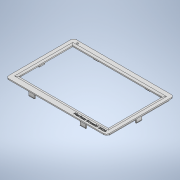
# Autodesk Inventor part: Top
Saved by Autodesk Inventor 2021 (Build 250183000, 183)
## iProperties
Created: 2020-06-15
Part Number: Top
Material: Generic
Document SubType Name: Modeling
Designer: Mariano
Density: 1 g/cm^3
Appearance: Default
Author: Mariano
Autodesk Inventor part; units mm, degrees
ref_plane "YZ Plane" through (0, 0, 0) normal (1, 0, 0) x (0, 1, 0)
ref_plane "XZ Plane" through (0, 0, 0) normal (0, 1, 0) x (-1, 0, 0)
ref_plane "XY Plane" through (0, 0, 0) normal (0, 0, 1) x (1, 0, 0)
sketch "Sketch1" plane through (0, 0, 0) normal (0, 1, 0) x (-1, 0, 0)
  line L0 (-92.2, 62) -> (92.2, 62)
  line L1 (92.2, 62) -> (92.2, -62)
  line L2 (92.2, -62) -> (-92.2, -62)
  line L3 (-92.2, -62) -> (-92.2, 62)
  line L4 (-92.2, 62) -> (92.2, -62) construction
  line L5 (92.2, 62) -> (-92.2, -62) construction
  line L6 (82.2, -50.5) -> (-82.2, -50.5)
  line L7 (-82.2, -50.5) -> (-82.2, 48.5)
  line L8 (-82.2, 48.5) -> (82.2, 48.5)
  line L9 (82.2, 48.5) -> (82.2, -50.5)
  line L10 (82.2, -50.5) -> (-82.2, 48.5) construction
  line L11 (-82.2, -50.5) -> (82.2, 48.5) construction
  line L12 (0, -62) -> (0, 62) construction
  line L13 (129.08, 0) -> (-129.08, 0) projected
  point P0 (0, 0)
  point P1 (0, -50.5)
  dimension "d2" = 184.4
  dimension "d3" = 124
  dimension "d34" = 164.4
  dimension "d35" = 99
  dimension "d50" = 13.5
  constraints: 26 end point, 5 midpoint, 5 perpendicular, 3 parallel, 1 point on line
  measures "d2" distance of L0.start L0.end
  measures "d3" distance of L0.end L1.end
  measures "d34" distance of L7.end L8.end
  measures "d35" distance of L6.end L7.end
  measures "d50" distance between parallel lines of L0 L8
extrude "Extrusion2" add sketch "Sketch1" along normal blind 3 contours L0 L1 L13 L9 L8 L7 L3 | L13 L7 L6 L9 L1 L2 L3
sketch "Sketch2" plane through (0, 0, 0) normal (0, -1, 0) x (1, 0, 0)
  line L0 (92.2, -62) -> (-92.2, -62) projected
  line L1 (-92.2, -62) -> (-92.2, 62) projected
  line L2 (92.2, -62) -> (-92.2, -62)
  line L3 (-92.2, -62) -> (-92.2, 62)
  line L4 (-92.2, 62) -> (92.2, 62)
  line L5 (92.2, 62) -> (92.2, -62)
  line L6 (90.2, -60) -> (-90.2, -60)
  line L7 (-90.2, -60) -> (-90.2, 60)
  line L8 (-90.2, 60) -> (90.2, 60)
  line L9 (90.2, 60) -> (90.2, -60)
  line L10 (0, -60) -> (0, 60)
  line L11 (-90.2, 0) -> (90.2, 0)
  point P0 (0, 0)
  dimension "d23" = 2
  constraints: 20 end point, 4 midpoint, 4 parallel, 2 perpendicular, 1 horizontal, 3 other
  measures "d23" distance between parallel lines of L9 L5
chamfer "Chamfer6" distance 4 distance2 1 1 edges at (-82.2, 3, -1) measured on face at (27.4, 3, 57.5)
chamfer "Chamfer7" distance 4 distance2 1 1 edges at (0, 3, -50.5) measured on face at (27.4, 3, 57.5)
chamfer "Chamfer8" distance 4 distance2 1 1 edges at (0, 3, 48.5) measured on face at (27.4, 3, 57.5)
chamfer "Chamfer9" distance 4 distance2 1 1 edges at (82.2, 3, -1) measured on face at (27.4, 3, 58.8333)
extrude "Extrusion5" cut sketch "Sketch2" against normal blind 1
fillet "Fillet1" radius 5 8 edges at (-92.2, 2, 62) (92.2, 2, 62) (-92.2, 2, -62) (92.2, 2, -62) (-90.2, 0.5, 60) (90.2, 0.5, 60) (90.2, 0.5, -60) (-90.2, 0.5, -60)
sketch "Sketch4" plane through (0, 0, 0) normal (0, -1, 0) x (1, 0, 0)
  line L0 (-85.2, -60) -> (85.2, -60) projected
  line L1 (52.2, -60) -> (42.2, -60)
  line L2 (42.2, -60) -> (42.2, -58)
  line L3 (42.2, -58) -> (52.2, -58)
  line L4 (52.2, -58) -> (52.2, -60)
  line L5 (92.2, 57) -> (92.2, -57) projected
  point P0 (0, 0)
  point P1 (42.2, -60)
  dimension "d53" = 10
  dimension "d54" = 2
  dimension "d55" = 40
  constraints: 8 end point, 2 parallel, 1 horizontal, 1 perpendicular, 1 point on line
  measures "d53" distance of L2.end L3.end
  measures "d54" distance of L1.end L2.end
  measures "d55" distance between parallel lines of L5 L4
extrude "Extrusion7" add sketch "Sketch4" along normal blind 8
chamfer "Chamfer10" distance 2 angle 45 2 edges at (42.2, 0, -59) (52.2, 0, -59)
chamfer "Chamfer11" distance 1 angle 45 1 edges at (47.2, 0, -58)
sketch "Sketch5" plane through (85.2, 1, -60) normal (0, 0, -1) x (-1, 0, 0)
  line L0 (33, -9) -> (43, -9) projected
  line L1 (33, -3) -> (33, -9) projected
  line L2 (43, -9) -> (33, -9)
  line L3 (33, -9) -> (33, -8)
  line L4 (33, -8) -> (43, -8)
  line L5 (43, -8) -> (43, -9)
  point P0 (85.2, -1)
  dimension "d64" = 1
  constraints: 8 end point, 2 parallel, 1 horizontal, 1 perpendicular, 1 point on line
  measures "d64" distance of L4.end L0.end
extrude "Extrusion8" add sketch "Sketch5" along normal blind 0.8
chamfer "Chamfer12" distance 1 distance2 0.8 1 edges at (47.2, -8, -60.8) measured on face at (45.5333, -7.6667, -60.8)
mirror "Mirror1" about plane through (0, 0, 0) normal (1, 0, 0) of "Extrusion7", "Chamfer10", "Chamfer11", "Extrusion8", "Chamfer12"
mirror "Mirror2" about plane through (0, 0, 0) normal (0, 0, 1) of "Extrusion7", "Chamfer10", "Chamfer11", "Extrusion8", "Chamfer12", "Mirror1"
sketch "Sketch6" plane through (0, 0, 0) normal (0, -1, 0) x (1, 0, 0)
  line L0 (-90.2, 55) -> (-90.2, -55) projected
  line L1 (-90.2, -5) -> (-88.2, -5)
  line L2 (-88.2, -5) -> (-88.2, 5)
  line L3 (-88.2, 5) -> (-90.2, 5)
  line L4 (-90.2, 5) -> (-90.2, -5)
  line L5 (87.2, -62) -> (-87.2, -62) projected
  line L6 (-129.08, 0) -> (129.08, 0) projected
  point P0 (0, 0)
  point P1 (-90.2, 0)
  dimension "d70" = 2
  dimension "d72" = 10
  constraints: 8 end point, 2 parallel, 2 point on line, 1 horizontal, 1 midpoint, 1 perpendicular
  measures "d70" distance of L3.end L2.end
  measures "d72" distance of L1.end L2.end
extrude "Extrusion9" add sketch "Sketch6" along normal blind 8
chamfer "Chamfer13" distance 2 angle 45 2 edges at (-89.2, 0, 5) (-89.2, 0, -5)
chamfer "Chamfer14" distance 1 angle 45 1 edges at (-88.2, 0, 0)
sketch "Sketch7" plane through (-90.2, 1, -55) normal (-1, 0, 0) x (0, 0, 1)
  line L0 (50, -9) -> (60, -9) projected
  line L1 (50, -3) -> (50, -9) projected
  line L2 (60, -9) -> (50, -9)
  line L3 (50, -9) -> (50, -8)
  line L4 (50, -8) -> (60, -8)
  line L5 (60, -8) -> (60, -9)
  point P0 (55, -1)
  dimension "d81" = 1
  constraints: 8 end point, 2 parallel, 1 horizontal, 1 perpendicular, 1 point on line
  measures "d81" distance between parallel lines of L4 L0
extrude "Extrusion10" add sketch "Sketch7" along normal blind 0.8
chamfer "Chamfer15" distance 1 distance2 0.8 1 edges at (-91, -8, 0) measured on face at (-91, -7.6667, 1.6667)
sketch "Sketch8" plane through (0, 3, 0) normal (0, 1, 0) x (1, 0, 0)
  circle A0 centre (-80, 57) radius 1.6
  line L0 (87.2, 62) -> (-87.2, 62) projected
  line L1 (-92.2, 57) -> (-92.2, -57) projected
  point P0 (0, 0)
  dimension "d87" = 3.2
  dimension "d95" = 5
  dimension "d96" = 12.2
  constraints: 1 centre point
  measures "d87" diameter of A0
  measures "d95" distance from line of L0 A0.centre
  measures "d96" distance from line of L1 A0.centre
extrude "Extrusion11" cut sketch "Sketch8" against normal through all
sketch "Sketch10" plane through (0, 3, 0) normal (0, 1, 0) x (1, 0, 0)
  line L0 (27.6834, -54.44) -> (87.3186, -54.44) construction
  line L1 (87.3186, -54.44) -> (87.3186, -59.4434) construction
  line L2 (87.3186, -59.4434) -> (27.6834, -59.4434) construction
  line L3 (27.6834, -59.4434) -> (27.6834, -54.44) construction
  line L4 (32.1826, -58.6216) -> (31.1842, -58.6216)
  line L5 (31.1842, -58.6216) -> (31.1842, -55.97)
  line L6 (31.1842, -55.97) -> (30.4581, -57.6815)
  line L7 (30.4581, -57.6815) -> (29.7709, -57.6815)
  line L8 (29.7709, -57.6815) -> (29.0448, -55.97)
  line L9 (29.0448, -55.97) -> (29.0448, -58.6216)
  line L10 (29.0448, -58.6216) -> (28.0983, -58.6216)
  line L11 (28.0983, -58.6216) -> (28.0983, -54.6216)
  line L12 (28.0983, -54.6216) -> (29.2555, -54.6216)
  line L13 (29.2555, -54.6216) -> (30.1437, -56.5956)
  line L14 (30.1437, -56.5956) -> (31.0254, -54.6216)
  line L15 (31.0254, -54.6216) -> (32.1826, -54.6216)
  line L16 (32.1826, -54.6216) -> (32.1826, -58.6216)
  spline S0 degree 2 poles (34.6202, -58.3007) (34.5229, -58.3817) (34.3706, -58.5114) (34.2409, -58.5762) knots 0 0 0 1 2 2 2
  spline S1 degree 2 poles (34.2409, -58.5762) (34.1145, -58.6378) (33.8746, -58.7026) (33.6607, -58.7026) knots 0 0 0 1 2 2 2
  spline S2 degree 2 poles (33.6607, -58.7026) (33.2588, -58.7026) (32.7304, -58.1645) (32.7304, -57.7561) knots 0 0 0 1 2 2 2
  spline S3 degree 2 poles (32.7304, -57.7561) (32.7304, -57.4222) (32.9994, -57.0073) (33.2523, -56.8874) knots 0 0 0 1 2 2 2
  spline S4 degree 2 poles (33.2523, -56.8874) (33.5084, -56.7642) (34.2182, -56.667) (34.6267, -56.641) knots 0 0 0 1 2 2 2
  line L17 (34.6267, -56.641) -> (34.6267, -56.6248)
  spline S5 degree 2 poles (34.6267, -56.6248) (34.6267, -56.3752) (34.2571, -56.184) (33.8876, -56.184) knots 0 0 0 1 2 2 2
  spline S6 degree 2 poles (33.8876, -56.184) (33.7223, -56.184) (33.275, -56.3039) (33.0643, -56.3979) knots 0 0 0 1 2 2 2
  line L18 (33.0643, -56.3979) -> (32.9832, -56.3979)
  line L19 (32.9832, -56.3979) -> (32.9832, -55.6686)
  spline S7 degree 2 poles (32.9832, -55.6686) (33.1226, -55.6297) (33.745, -55.5195) (34.0627, -55.5195) knots 0 0 0 1 2 2 2
  spline S8 degree 2 poles (34.0627, -55.5195) (34.8406, -55.5195) (35.5537, -56.0381) (35.5537, -56.5697) knots 0 0 0 1 2 2 2
  line L20 (35.5537, -56.5697) -> (35.5537, -58.6216)
  line L21 (35.5537, -58.6216) -> (34.6202, -58.6216)
  line L22 (34.6202, -58.6216) -> (34.6202, -58.3007)
  line L23 (34.6202, -57.8339) -> (34.6202, -57.2083)
  spline S9 degree 2 poles (34.6202, -57.2083) (34.3803, -57.231) (34.0853, -57.2666) (33.9427, -57.3185) knots 0 0 0 1 2 2 2
  spline S10 degree 2 poles (33.9427, -57.3185) (33.8163, -57.3606) (33.6802, -57.5357) (33.6802, -57.6783) knots 0 0 0 1 2 2 2
  spline S11 degree 2 poles (33.6802, -57.6783) (33.6802, -57.889) (33.9103, -58.0478) (34.134, -58.0478) knots 0 0 0 1 2 2 2
  spline S12 degree 2 poles (34.134, -58.0478) (34.2571, -58.0478) (34.5165, -57.9344) (34.6202, -57.8339) knots 0 0 0 1 2 2 2
  line L24 (38.2766, -56.4952) -> (38.1988, -56.4952)
  spline S13 degree 2 poles (38.1988, -56.4952) (38.1437, -56.4757) (37.9395, -56.4563) (37.8163, -56.4563) knots 0 0 0 1 2 2 2
  spline S14 degree 2 poles (37.8163, -56.4563) (37.6704, -56.4563) (37.343, -56.5438) (37.1907, -56.6021) knots 0 0 0 1 2 2 2
  line L25 (37.1907, -56.6021) -> (37.1907, -58.6216)
  line L26 (37.1907, -58.6216) -> (36.2507, -58.6216)
  line L27 (36.2507, -58.6216) -> (36.2507, -55.6037)
  line L28 (36.2507, -55.6037) -> (37.1907, -55.6037)
  line L29 (37.1907, -55.6037) -> (37.1907, -56.0381)
  spline S15 degree 2 poles (37.1907, -56.0381) (37.2555, -55.9798) (37.4824, -55.7982) (37.5764, -55.7431) knots 0 0 0 1 2 2 2
  spline S16 degree 2 poles (37.5764, -55.7431) (37.6802, -55.6815) (37.9524, -55.594) (38.0724, -55.594) knots 0 0 0 1 2 2 2
  spline S17 degree 2 poles (38.0724, -55.594) (38.1178, -55.594) (38.2312, -55.6005) (38.2766, -55.6037) knots 0 0 0 1 2 2 2
  line L30 (38.2766, -55.6037) -> (38.2766, -56.4952)
  line L31 (39.5764, -58.6216) -> (38.6364, -58.6216)
  line L32 (38.6364, -58.6216) -> (38.6364, -55.6037)
  line L33 (38.6364, -55.6037) -> (39.5764, -55.6037)
  line L34 (39.5764, -55.6037) -> (39.5764, -58.6216)
  line L35 (39.6056, -55.1726) -> (38.6105, -55.1726)
  line L36 (38.6105, -55.1726) -> (38.6105, -54.44)
  line L37 (38.6105, -54.44) -> (39.6056, -54.44)
  line L38 (39.6056, -54.44) -> (39.6056, -55.1726)
  line L39 (43.0967, -58.6216) -> (42.1567, -58.6216)
  line L40 (42.1567, -58.6216) -> (42.1567, -58.2877)
  spline S18 degree 2 poles (42.1567, -58.2877) (41.9135, -58.4919) (41.5051, -58.7059) (41.2231, -58.7059) knots 0 0 0 1 2 2 2
  spline S19 degree 2 poles (41.2231, -58.7059) (40.7758, -58.7059) (40.2733, -58.1386) (40.2733, -57.5681) knots 0 0 0 1 2 2 2
  line L41 (40.2733, -57.5681) -> (40.2733, -55.6037)
  line L42 (40.2733, -55.6037) -> (41.2199, -55.6037)
  line L43 (41.2199, -55.6037) -> (41.2199, -57.1013)
  spline S20 degree 2 poles (41.2199, -57.1013) (41.2199, -57.3347) (41.2426, -57.6329) (41.2879, -57.7334) knots 0 0 0 1 2 2 2
  spline S21 degree 2 poles (41.2879, -57.7334) (41.3333, -57.8274) (41.5116, -57.9247) (41.6737, -57.9247) knots 0 0 0 1 2 2 2
  spline S22 degree 2 poles (41.6737, -57.9247) (41.7709, -57.9247) (42.0432, -57.8274) (42.1567, -57.7431) knots 0 0 0 1 2 2 2
  line L44 (42.1567, -57.7431) -> (42.1567, -55.6037)
  line L45 (42.1567, -55.6037) -> (43.0967, -55.6037)
  line L46 (43.0967, -55.6037) -> (43.0967, -58.6216)
  spline S23 degree 2 poles (44.7336, -58.7026) (44.403, -58.7026) (43.8098, -58.5567) (43.6153, -58.4595) knots 0 0 0 1 2 2 2
  line L47 (43.6153, -58.4595) -> (43.6153, -57.6653)
  line L48 (43.6153, -57.6653) -> (43.6931, -57.6653)
  spline S24 degree 2 poles (43.6931, -57.6653) (43.7612, -57.7172) (43.933, -57.8404) (44.0853, -57.9084) knots 0 0 0 1 2 2 2
  spline S25 degree 2 poles (44.0853, -57.9084) (44.2182, -57.97) (44.5456, -58.0576) (44.7401, -58.0576) knots 0 0 0 1 2 2 2
  spline S26 degree 2 poles (44.7401, -58.0576) (44.9379, -58.0576) (45.2426, -57.9344) (45.2426, -57.8015) knots 0 0 0 1 2 2 2
  spline S27 degree 2 poles (45.2426, -57.8015) (45.2426, -57.6977) (45.1032, -57.5875) (44.9022, -57.5422) knots 0 0 0 1 2 2 2
  spline S28 degree 2 poles (44.9022, -57.5422) (44.7952, -57.513) (44.4678, -57.4514) (44.3414, -57.4125) knots 0 0 0 1 2 2 2
  spline S29 degree 2 poles (44.3414, -57.4125) (43.9849, -57.3023) (43.6283, -56.8712) (43.6283, -56.5178) knots 0 0 0 1 2 2 2
  spline S30 degree 2 poles (43.6283, -56.5178) (43.6283, -56.3169) (43.8131, -55.9603) (43.9946, -55.8209) knots 0 0 0 1 2 2 2
  spline S31 degree 2 poles (43.9946, -55.8209) (44.1729, -55.6848) (44.7012, -55.5227) (45.0351, -55.5227) knots 0 0 0 1 2 2 2
  spline S32 degree 2 poles (45.0351, -55.5227) (45.3528, -55.5227) (45.8844, -55.6491) (46.0659, -55.7366) knots 0 0 0 1 2 2 2
  line L49 (46.0659, -55.7366) -> (46.0659, -56.5016)
  line L50 (46.0659, -56.5016) -> (45.9913, -56.5016)
  spline S33 degree 2 poles (45.9913, -56.5016) (45.9427, -56.4627) (45.732, -56.3363) (45.6348, -56.2909) knots 0 0 0 1 2 2 2
  spline S34 degree 2 poles (45.6348, -56.2909) (45.5148, -56.2391) (45.2231, -56.1678) (45.0708, -56.1678) knots 0 0 0 1 2 2 2
  spline S35 degree 2 poles (45.0708, -56.1678) (44.8665, -56.1678) (44.5845, -56.3071) (44.5845, -56.4206) knots 0 0 0 1 2 2 2
  spline S36 degree 2 poles (44.5845, -56.4206) (44.5845, -56.5243) (44.7239, -56.641) (44.9573, -56.6994) knots 0 0 0 1 2 2 2
  spline S37 degree 2 poles (44.9573, -56.6994) (45.0772, -56.7285) (45.3917, -56.7836) (45.5375, -56.8323) knots 0 0 0 1 2 2 2
  spline S38 degree 2 poles (45.5375, -56.8323) (45.8617, -56.936) (46.1988, -57.3412) (46.1988, -57.6783) knots 0 0 0 1 2 2 2
  spline S39 degree 2 poles (46.1988, -57.6783) (46.1988, -57.889) (46.0011, -58.2747) (45.8163, -58.4044) knots 0 0 0 1 2 2 2
  spline S40 degree 2 poles (45.8163, -58.4044) (45.6251, -58.547) (45.0999, -58.7026) (44.7336, -58.7026) knots 0 0 0 1 2 2 2
  line L51 (49.0513, -58.6216) -> (46.416, -58.6216)
  line L52 (46.416, -58.6216) -> (46.416, -58.0024)
  line L53 (46.416, -58.0024) -> (47.8552, -56.3104)
  line L54 (47.8552, -56.3104) -> (46.4808, -56.3104)
  line L55 (46.4808, -56.3104) -> (46.4808, -55.6037)
  line L56 (46.4808, -55.6037) -> (49.0221, -55.6037)
  line L57 (49.0221, -55.6037) -> (49.0221, -56.2131)
  line L58 (49.0221, -56.2131) -> (47.5797, -57.902)
  line L59 (47.5797, -57.902) -> (49.0513, -57.902)
  line L60 (49.0513, -57.902) -> (49.0513, -58.6216)
  spline S41 degree 2 poles (54.3998, -57.3963) (54.3998, -57.6945) (54.1729, -58.1451) (53.9849, -58.2942) knots 0 0 0 1 2 2 2
  spline S42 degree 2 poles (53.9849, -58.2942) (53.758, -58.4725) (53.2199, -58.6216) (52.8017, -58.6216) knots 0 0 0 1 2 2 2
  line L61 (52.8017, -58.6216) -> (51.2037, -58.6216)
  line L62 (51.2037, -58.6216) -> (51.2037, -54.6216)
  line L63 (51.2037, -54.6216) -> (52.6137, -54.6216)
  spline S43 degree 2 poles (52.6137, -54.6216) (53.0545, -54.6216) (53.5084, -54.6896) (53.7061, -54.7966) knots 0 0 0 1 2 2 2
  spline S44 degree 2 poles (53.7061, -54.7966) (53.9233, -54.9101) (54.134, -55.299) (54.134, -55.5519) knots 0 0 0 1 2 2 2
  spline S45 degree 2 poles (54.134, -55.5519) (54.134, -55.8436) (53.8422, -56.3007) (53.5829, -56.4076) knots 0 0 0 1 2 2 2
  line L64 (53.5829, -56.4076) -> (53.5829, -56.4271)
  spline S46 degree 2 poles (53.5829, -56.4271) (53.9557, -56.5049) (54.3998, -56.9879) (54.3998, -57.3963) knots 0 0 0 1 2 2 2
  spline S47 degree 2 poles (53.3625, -57.3801) (53.3625, -57.1921) (53.2134, -56.9814) (53.0643, -56.9263) knots 0 0 0 1 2 2 2
  spline S48 degree 2 poles (53.0643, -56.9263) (52.9735, -56.8906) (52.6526, -56.8841) (52.3868, -56.8841) knots 0 0 0 1 2 2 2
  line L65 (52.3868, -56.8841) -> (52.202, -56.8841)
  line L66 (52.202, -56.8841) -> (52.202, -57.8922)
  line L67 (52.202, -57.8922) -> (52.2571, -57.8922)
  spline S49 degree 2 poles (52.2571, -57.8922) (52.6461, -57.8922) (52.9443, -57.8825) (53.0999, -57.8144) knots 0 0 0 1 2 2 2
  spline S50 degree 2 poles (53.0999, -57.8144) (53.2361, -57.7529) (53.3625, -57.5259) (53.3625, -57.3801) knots 0 0 0 1 2 2 2
  spline S51 degree 2 poles (53.1129, -55.7496) (53.1129, -55.6524) (53.0124, -55.4482) (52.9087, -55.4028) knots 0 0 0 1 2 2 2
  spline S52 degree 2 poles (52.9087, -55.4028) (52.8114, -55.3574) (52.5392, -55.3509) (52.2701, -55.3509) knots 0 0 0 1 2 2 2
  line L68 (52.2701, -55.3509) -> (52.202, -55.3509)
  line L69 (52.202, -55.3509) -> (52.202, -56.2002)
  line L70 (52.202, -56.2002) -> (52.3285, -56.2002)
  spline S53 degree 2 poles (52.3285, -56.2002) (52.5845, -56.2002) (52.792, -56.1905) (52.9022, -56.1386) knots 0 0 0 1 2 2 2
  spline S54 degree 2 poles (52.9022, -56.1386) (53.0221, -56.0802) (53.1129, -55.8825) (53.1129, -55.7496) knots 0 0 0 1 2 2 2
  line L71 (56.9476, -56.4952) -> (56.8698, -56.4952)
  spline S55 degree 2 poles (56.8698, -56.4952) (56.8147, -56.4757) (56.6105, -56.4563) (56.4873, -56.4563) knots 0 0 0 1 2 2 2
  spline S56 degree 2 poles (56.4873, -56.4563) (56.3414, -56.4563) (56.014, -56.5438) (55.8617, -56.6021) knots 0 0 0 1 2 2 2
  line L72 (55.8617, -56.6021) -> (55.8617, -58.6216)
  line L73 (55.8617, -58.6216) -> (54.9216, -58.6216)
  line L74 (54.9216, -58.6216) -> (54.9216, -55.6037)
  line L75 (54.9216, -55.6037) -> (55.8617, -55.6037)
  line L76 (55.8617, -55.6037) -> (55.8617, -56.0381)
  spline S57 degree 2 poles (55.8617, -56.0381) (55.9265, -55.9798) (56.1534, -55.7982) (56.2474, -55.7431) knots 0 0 0 1 2 2 2
  spline S58 degree 2 poles (56.2474, -55.7431) (56.3511, -55.6815) (56.6234, -55.594) (56.7434, -55.594) knots 0 0 0 1 2 2 2
  spline S59 degree 2 poles (56.7434, -55.594) (56.7887, -55.594) (56.9022, -55.6005) (56.9476, -55.6037) knots 0 0 0 1 2 2 2
  line L77 (56.9476, -55.6037) -> (56.9476, -56.4952)
  line L78 (59.7126, -58.6216) -> (57.0772, -58.6216)
  line L79 (57.0772, -58.6216) -> (57.0772, -58.0024)
  line L80 (57.0772, -58.0024) -> (58.5165, -56.3104)
  line L81 (58.5165, -56.3104) -> (57.1421, -56.3104)
  line L82 (57.1421, -56.3104) -> (57.1421, -55.6037)
  line L83 (57.1421, -55.6037) -> (59.6834, -55.6037)
  line L84 (59.6834, -55.6037) -> (59.6834, -56.2131)
  line L85 (59.6834, -56.2131) -> (58.2409, -57.902)
  line L86 (58.2409, -57.902) -> (59.7126, -57.902)
  line L87 (59.7126, -57.902) -> (59.7126, -58.6216)
  spline S60 degree 2 poles (61.745, -58.7026) (60.8892, -58.7026) (59.9784, -57.8858) (59.9784, -57.1305) knots 0 0 0 1 2 2 2
  spline S61 degree 2 poles (59.9784, -57.1305) (59.9784, -56.3914) (60.8276, -55.5097) (61.5926, -55.5097) knots 0 0 0 1 2 2 2
  spline S62 degree 2 poles (61.5926, -55.5097) (62.2831, -55.5097) (62.9832, -56.2585) (62.9832, -56.9522) knots 0 0 0 1 2 2 2
  line L88 (62.9832, -56.9522) -> (62.9832, -57.2926)
  line L89 (62.9832, -57.2926) -> (60.9184, -57.2926)
  spline S63 degree 2 poles (60.9184, -57.2926) (60.9314, -57.5033) (61.0837, -57.782) (61.2069, -57.8663) knots 0 0 0 1 2 2 2
  spline S64 degree 2 poles (61.2069, -57.8663) (61.3268, -57.9506) (61.651, -58.0219) (61.8422, -58.0219) knots 0 0 0 1 2 2 2
  spline S65 degree 2 poles (61.8422, -58.0219) (62.0043, -58.0219) (62.322, -57.9506) (62.4549, -57.889) knots 0 0 0 1 2 2 2
  spline S66 degree 2 poles (62.4549, -57.889) (62.5716, -57.8404) (62.7661, -57.7204) (62.8276, -57.6751) knots 0 0 0 1 2 2 2
  line L90 (62.8276, -57.6751) -> (62.9281, -57.6751)
  line L91 (62.9281, -57.6751) -> (62.9281, -58.453)
  spline S67 degree 2 poles (62.9281, -58.453) (62.8114, -58.4984) (62.6234, -58.5762) (62.4549, -58.6151) knots 0 0 0 1 2 2 2
  spline S68 degree 2 poles (62.4549, -58.6151) (62.3025, -58.6572) (61.9784, -58.7026) (61.745, -58.7026) knots 0 0 0 1 2 2 2
  spline S69 degree 2 poles (62.0562, -56.7253) (62.0497, -56.4271) (61.7871, -56.1127) (61.5181, -56.1127) knots 0 0 0 1 2 2 2
  spline S70 degree 2 poles (61.5181, -56.1127) (61.2426, -56.1127) (60.9314, -56.4433) (60.9152, -56.7253) knots 0 0 0 1 2 2 2
  line L92 (60.9152, -56.7253) -> (62.0562, -56.7253)
  spline S71 degree 2 poles (64.3836, -58.7026) (64.0529, -58.7026) (63.4597, -58.5567) (63.2652, -58.4595) knots 0 0 0 1 2 2 2
  line L93 (63.2652, -58.4595) -> (63.2652, -57.6653)
  line L94 (63.2652, -57.6653) -> (63.343, -57.6653)
  spline S72 degree 2 poles (63.343, -57.6653) (63.4111, -57.7172) (63.5829, -57.8404) (63.7353, -57.9084) knots 0 0 0 1 2 2 2
  spline S73 degree 2 poles (63.7353, -57.9084) (63.8682, -57.97) (64.1956, -58.0576) (64.39, -58.0576) knots 0 0 0 1 2 2 2
  spline S74 degree 2 poles (64.39, -58.0576) (64.5878, -58.0576) (64.8925, -57.9344) (64.8925, -57.8015) knots 0 0 0 1 2 2 2
  spline S75 degree 2 poles (64.8925, -57.8015) (64.8925, -57.6977) (64.7531, -57.5875) (64.5521, -57.5422) knots 0 0 0 1 2 2 2
  spline S76 degree 2 poles (64.5521, -57.5422) (64.4451, -57.513) (64.1178, -57.4514) (63.9913, -57.4125) knots 0 0 0 1 2 2 2
  spline S77 degree 2 poles (63.9913, -57.4125) (63.6348, -57.3023) (63.2782, -56.8712) (63.2782, -56.5178) knots 0 0 0 1 2 2 2
  spline S78 degree 2 poles (63.2782, -56.5178) (63.2782, -56.3169) (63.463, -55.9603) (63.6445, -55.8209) knots 0 0 0 1 2 2 2
  spline S79 degree 2 poles (63.6445, -55.8209) (63.8228, -55.6848) (64.3511, -55.5227) (64.685, -55.5227) knots 0 0 0 1 2 2 2
  spline S80 degree 2 poles (64.685, -55.5227) (65.0027, -55.5227) (65.5343, -55.6491) (65.7158, -55.7366) knots 0 0 0 1 2 2 2
  line L95 (65.7158, -55.7366) -> (65.7158, -56.5016)
  line L96 (65.7158, -56.5016) -> (65.6413, -56.5016)
  spline S81 degree 2 poles (65.6413, -56.5016) (65.5926, -56.4627) (65.3819, -56.3363) (65.2847, -56.2909) knots 0 0 0 1 2 2 2
  spline S82 degree 2 poles (65.2847, -56.2909) (65.1648, -56.2391) (64.873, -56.1678) (64.7207, -56.1678) knots 0 0 0 1 2 2 2
  spline S83 degree 2 poles (64.7207, -56.1678) (64.5165, -56.1678) (64.2345, -56.3071) (64.2345, -56.4206) knots 0 0 0 1 2 2 2
  spline S84 degree 2 poles (64.2345, -56.4206) (64.2345, -56.5243) (64.3738, -56.641) (64.6072, -56.6994) knots 0 0 0 1 2 2 2
  spline S85 degree 2 poles (64.6072, -56.6994) (64.7272, -56.7285) (65.0416, -56.7836) (65.1875, -56.8323) knots 0 0 0 1 2 2 2
  spline S86 degree 2 poles (65.1875, -56.8323) (65.5116, -56.936) (65.8487, -57.3412) (65.8487, -57.6783) knots 0 0 0 1 2 2 2
  spline S87 degree 2 poles (65.8487, -57.6783) (65.8487, -57.889) (65.651, -58.2747) (65.4662, -58.4044) knots 0 0 0 1 2 2 2
  spline S88 degree 2 poles (65.4662, -58.4044) (65.275, -58.547) (64.7498, -58.7026) (64.3836, -58.7026) knots 0 0 0 1 2 2 2
  line L97 (69.3171, -58.6216) -> (68.1988, -58.6216)
  line L98 (68.1988, -58.6216) -> (67.3819, -57.312)
  line L99 (67.3819, -57.312) -> (67.2361, -57.5065)
  line L100 (67.2361, -57.5065) -> (67.2361, -58.6216)
  line L101 (67.2361, -58.6216) -> (66.296, -58.6216)
  line L102 (66.296, -58.6216) -> (66.296, -54.4433)
  line L103 (66.296, -54.4433) -> (67.2361, -54.4433)
  line L104 (67.2361, -54.4433) -> (67.2361, -56.7836)
  line L105 (67.2361, -56.7836) -> (68.1275, -55.6037)
  line L106 (68.1275, -55.6037) -> (69.2393, -55.6037)
  line L107 (69.2393, -55.6037) -> (68.1826, -56.9036)
  line L108 (68.1826, -56.9036) -> (69.3171, -58.6216)
  line L109 (70.5521, -58.6216) -> (69.6121, -58.6216)
  line L110 (69.6121, -58.6216) -> (69.6121, -55.6037)
  line L111 (69.6121, -55.6037) -> (70.5521, -55.6037)
  line L112 (70.5521, -55.6037) -> (70.5521, -58.6216)
  line L113 (70.5813, -55.1726) -> (69.5862, -55.1726)
  line L114 (69.5862, -55.1726) -> (69.5862, -54.44)
  line L115 (69.5862, -54.44) -> (70.5813, -54.44)
  line L116 (70.5813, -54.44) -> (70.5813, -55.1726)
  line L117 (75.8682, -58.6216) -> (72.9281, -58.6216)
  line L118 (72.9281, -58.6216) -> (72.9281, -57.97)
  spline S89 degree 2 poles (72.9281, -57.97) (73.3009, -57.6718) (73.8973, -57.1467) (74.121, -56.9101) knots 0 0 0 1 2 2 2
  spline S90 degree 2 poles (74.121, -56.9101) (74.416, -56.6021) (74.6785, -56.1321) (74.6785, -55.8858) knots 0 0 0 1 2 2 2
  spline S91 degree 2 poles (74.6785, -55.8858) (74.6785, -55.607) (74.3447, -55.3088) (74.0464, -55.3088) knots 0 0 0 1 2 2 2
  spline S92 degree 2 poles (74.0464, -55.3088) (73.8941, -55.3088) (73.6218, -55.3833) (73.4824, -55.4417) knots 0 0 0 1 2 2 2
  spline S93 degree 2 poles (73.4824, -55.4417) (73.3463, -55.5033) (73.1518, -55.6329) (73.1032, -55.6653) knots 0 0 0 1 2 2 2
  line L119 (73.1032, -55.6653) -> (73.0254, -55.6653)
  line L120 (73.0254, -55.6653) -> (73.0254, -54.7934)
  spline S94 degree 2 poles (73.0254, -54.7934) (73.1939, -54.7123) (73.9135, -54.5438) (74.2474, -54.5438) knots 0 0 0 1 2 2 2
  spline S95 degree 2 poles (74.2474, -54.5438) (74.9605, -54.5438) (75.6931, -55.1791) (75.6931, -55.7529) knots 0 0 0 1 2 2 2
  spline S96 degree 2 poles (75.6931, -55.7529) (75.6931, -56.1062) (75.3592, -56.7869) (74.9735, -57.1759) knots 0 0 0 1 2 2 2
  spline S97 degree 2 poles (74.9735, -57.1759) (74.7304, -57.4157) (74.2734, -57.7885) (74.1729, -57.8663) knots 0 0 0 1 2 2 2
  line L121 (74.1729, -57.8663) -> (75.8682, -57.8663)
  line L122 (75.8682, -57.8663) -> (75.8682, -58.6216)
  spline S98 degree 2 poles (79.3204, -56.6216) (79.3204, -57.1402) (79.155, -57.9182) (78.9703, -58.1807) knots 0 0 0 1 2 2 2
  spline S99 degree 2 poles (78.9703, -58.1807) (78.7887, -58.44) (78.202, -58.7059) (77.7806, -58.7059) knots 0 0 0 1 2 2 2
  spline S100 degree 2 poles (77.7806, -58.7059) (77.356, -58.7059) (76.7725, -58.44) (76.5878, -58.1742) knots 0 0 0 1 2 2 2
  spline S101 degree 2 poles (76.5878, -58.1742) (76.403, -57.9117) (76.2377, -57.1402) (76.2377, -56.6216) knots 0 0 0 1 2 2 2
  spline S102 degree 2 poles (76.2377, -56.6216) (76.2377, -56.09) (76.403, -55.3379) (76.591, -55.0657) knots 0 0 0 1 2 2 2
  spline S103 degree 2 poles (76.591, -55.0657) (76.779, -54.7999) (77.3722, -54.5405) (77.7806, -54.5405) knots 0 0 0 1 2 2 2
  spline S104 degree 2 poles (77.7806, -54.5405) (78.2118, -54.5405) (78.7887, -54.8128) (78.9735, -55.0819) knots 0 0 0 1 2 2 2
  spline S105 degree 2 poles (78.9735, -55.0819) (79.155, -55.3444) (79.3204, -56.1191) (79.3204, -56.6216) knots 0 0 0 1 2 2 2
  spline S106 degree 2 poles (78.3122, -56.6216) (78.3122, -55.8793) (78.0691, -55.2796) (77.7806, -55.2796) knots 0 0 0 1 2 2 2
  spline S107 degree 2 poles (77.7806, -55.2796) (77.4922, -55.2796) (77.2458, -55.8793) (77.2458, -56.6248) knots 0 0 0 1 2 2 2
  spline S108 degree 2 poles (77.2458, -56.6248) (77.2458, -57.3574) (77.4922, -57.9668) (77.7806, -57.9668) knots 0 0 0 1 2 2 2
  spline S109 degree 2 poles (77.7806, -57.9668) (78.0659, -57.9668) (78.3122, -57.3574) (78.3122, -56.6216) knots 0 0 0 1 2 2 2
  line L123 (82.8763, -58.6216) -> (79.9362, -58.6216)
  line L124 (79.9362, -58.6216) -> (79.9362, -57.97)
  spline S110 degree 2 poles (79.9362, -57.97) (80.309, -57.6718) (80.9054, -57.1467) (81.1291, -56.9101) knots 0 0 0 1 2 2 2
  spline S111 degree 2 poles (81.1291, -56.9101) (81.4241, -56.6021) (81.6866, -56.1321) (81.6866, -55.8858) knots 0 0 0 1 2 2 2
  spline S112 degree 2 poles (81.6866, -55.8858) (81.6866, -55.607) (81.3528, -55.3088) (81.0545, -55.3088) knots 0 0 0 1 2 2 2
  spline S113 degree 2 poles (81.0545, -55.3088) (80.9022, -55.3088) (80.6299, -55.3833) (80.4905, -55.4417) knots 0 0 0 1 2 2 2
  spline S114 degree 2 poles (80.4905, -55.4417) (80.3544, -55.5033) (80.1599, -55.6329) (80.1113, -55.6653) knots 0 0 0 1 2 2 2
  line L125 (80.1113, -55.6653) -> (80.0335, -55.6653)
  line L126 (80.0335, -55.6653) -> (80.0335, -54.7934)
  spline S115 degree 2 poles (80.0335, -54.7934) (80.202, -54.7123) (80.9216, -54.5438) (81.2555, -54.5438) knots 0 0 0 1 2 2 2
  spline S116 degree 2 poles (81.2555, -54.5438) (81.9686, -54.5438) (82.7012, -55.1791) (82.7012, -55.7529) knots 0 0 0 1 2 2 2
  spline S117 degree 2 poles (82.7012, -55.7529) (82.7012, -56.1062) (82.3674, -56.7869) (81.9816, -57.1759) knots 0 0 0 1 2 2 2
  spline S118 degree 2 poles (81.9816, -57.1759) (81.7385, -57.4157) (81.2815, -57.7885) (81.181, -57.8663) knots 0 0 0 1 2 2 2
  line L127 (81.181, -57.8663) -> (82.8763, -57.8663)
  line L128 (82.8763, -57.8663) -> (82.8763, -58.6216)
  spline S119 degree 2 poles (86.3285, -56.6216) (86.3285, -57.1402) (86.1631, -57.9182) (85.9784, -58.1807) knots 0 0 0 1 2 2 2
  spline S120 degree 2 poles (85.9784, -58.1807) (85.7969, -58.44) (85.2101, -58.7059) (84.7887, -58.7059) knots 0 0 0 1 2 2 2
  spline S121 degree 2 poles (84.7887, -58.7059) (84.3641, -58.7059) (83.7806, -58.44) (83.5959, -58.1742) knots 0 0 0 1 2 2 2
  spline S122 degree 2 poles (83.5959, -58.1742) (83.4111, -57.9117) (83.2458, -57.1402) (83.2458, -56.6216) knots 0 0 0 1 2 2 2
  spline S123 degree 2 poles (83.2458, -56.6216) (83.2458, -56.09) (83.4111, -55.3379) (83.5991, -55.0657) knots 0 0 0 1 2 2 2
  spline S124 degree 2 poles (83.5991, -55.0657) (83.7871, -54.7999) (84.3803, -54.5405) (84.7887, -54.5405) knots 0 0 0 1 2 2 2
  spline S125 degree 2 poles (84.7887, -54.5405) (85.2199, -54.5405) (85.7969, -54.8128) (85.9816, -55.0819) knots 0 0 0 1 2 2 2
  spline S126 degree 2 poles (85.9816, -55.0819) (86.1631, -55.3444) (86.3285, -56.1191) (86.3285, -56.6216) knots 0 0 0 1 2 2 2
  spline S127 degree 2 poles (85.3204, -56.6216) (85.3204, -55.8793) (85.0772, -55.2796) (84.7887, -55.2796) knots 0 0 0 1 2 2 2
  spline S128 degree 2 poles (84.7887, -55.2796) (84.5003, -55.2796) (84.2539, -55.8793) (84.2539, -56.6248) knots 0 0 0 1 2 2 2
  spline S129 degree 2 poles (84.2539, -56.6248) (84.2539, -57.3574) (84.5003, -57.9668) (84.7887, -57.9668) knots 0 0 0 1 2 2 2
  spline S130 degree 2 poles (84.7887, -57.9668) (85.074, -57.9668) (85.3204, -57.3574) (85.3204, -56.6216) knots 0 0 0 1 2 2 2
  point P0 (0, 0)
  constraints: 2 other
extrude "Extrusion13" cut sketch "Sketch10" against normal blind 0.4
mirror "Mirror5" about plane through (0, 0, 0) normal (1, 0, 0) of "Chamfer15", "Extrusion10", "Chamfer14", "Chamfer13", "Extrusion9"
sketch "Sketch11" plane through (0, 0, 0) normal (0, -1, 0) x (1, 0, 0)
  line L0 (-90.2, 55) -> (-90.2, -55) projected
  line L1 (-90.2, 55) -> (-88.2, 55)
  line L2 (-88.2, 55) -> (-88.2, -55)
  line L3 (-88.2, -55) -> (-90.2, -55)
  line L4 (-90.2, -55) -> (-90.2, 55)
  line L5 (90.2, -55) -> (90.2, 55) projected
  line L6 (90.2, 55) -> (88.2, 55)
  line L7 (88.2, 55) -> (88.2, -55)
  line L8 (88.2, -55) -> (90.2, -55)
  line L9 (90.2, -55) -> (90.2, 55)
  line L10 (-85.2, -60) -> (85.2, -60) projected
  line L11 (-74, -58) -> (79, -58)
  line L12 (79, -58) -> (79, -60)
  line L13 (79, -60) -> (-74, -60)
  line L14 (-74, -60) -> (-74, -58)
  point P0 (0, 0)
  point P1 (-90.2, -55)
  dimension "d97" = 2
  dimension "d98" = 2
  dimension "d101" = 2
  constraints: 24 end point, 6 parallel, 3 horizontal, 3 perpendicular, 2 point on line
  measures "d97" distance of L2.end L3.end
  measures "d98" distance of L8.end L7.end
  measures "d101" distance of L11.end L12.end
extrude "Extrusion14" add sketch "Sketch11" along normal blind 2
body "Solid2"
